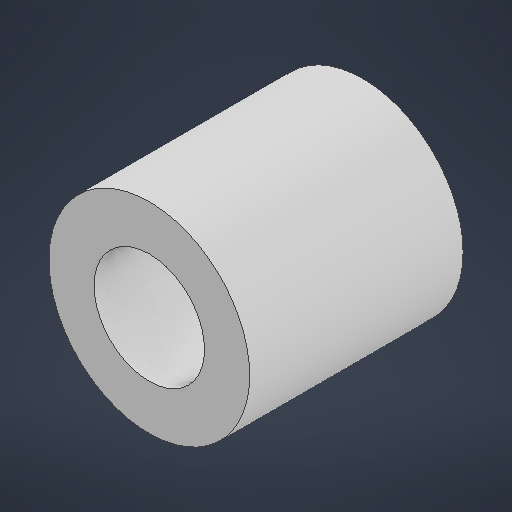
# Autodesk Inventor part: CH3-DiffBoxSpacersTop
Saved by Autodesk Inventor 2026.1 (Build 301233020, 233B)
## iProperties
Created: 2025-10-23
Part Number: CH3-DiffBoxSpacersTop
Material: Generic
Document SubType Name: Modeling
Designer: johnh
Density: 1 g/cm^3
Appearance: Default
Author: johnh
Autodesk Inventor part; units mm, degrees
ref_plane "YZ Plane" through (0, 0, 0) normal (1, 0, 0) x (0, 1, 0)
ref_plane "XZ Plane" through (0, 0, 0) normal (0, 1, 0) x (-1, 0, 0)
ref_plane "XY Plane" through (0, 0, 0) normal (0, 0, 1) x (1, 0, 0)
sketch "Sketch1" plane through (0, 0, 0) normal (0, 0, 1) x (1, 0, 0)
  circle A0 centre (0, 0) radius 12.7
  circle A1 centre (0, 0) radius 6.985
  dimension "d0" = 13.97
  dimension "d2" = 25.4
  constraints: 2 centre point, 1 coincident
  measures "d0" diameter of A1
  measures "d2" diameter of A0
extrude "Extrusion1" add sketch "Sketch1" against normal blind 27.0002
body "Solid1"
